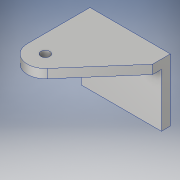
# Autodesk Inventor part: LeftAngleBracket-1111-2018
Saved by Autodesk Inventor 2017 (Build 210142000, 142)
## iProperties
Created: 2018-02-10
Part Number: LeftAngleBracket-1111-2018
Material: Aluminum 6061
Document SubType Name: Modeling
Designer: Phyllis
Density: 2.7 g/cm^3
Appearance: Aluminum - Flat
Author: Phyllis
Autodesk Inventor part; units mm, degrees
ref_plane "YZ Plane" through (0, 0, 0) normal (1, 0, 0) x (0, 1, 0)
ref_plane "XZ Plane" through (0, 0, 0) normal (0, 1, 0) x (-1, 0, 0)
ref_plane "XY Plane" through (0, 0, 0) normal (0, 0, 1) x (1, 0, 0)
sketch "Sketch1" plane through (0, 0, 0) normal (0, 0, 1) x (1, 0, 0)
  line L0 (0, 0) -> (28.575, 0)
  line L1 (28.575, 0) -> (28.575, 19.05)
  line L2 (28.575, 19.05) -> (0, 19.05)
  line L3 (0, 19.05) -> (0, 0)
  dimension "d4" = 28.575
  dimension "d5" = 19.05
  constraints: 8 end point, 2 parallel, 1 horizontal, 1 perpendicular
  measures "d4" distance of L0.start L0.end
  measures "d5" distance of L0.end L1.end
extrude "Extrusion1" add sketch "Sketch1" along normal blind 3.175
sketch "Sketch3" plane through (0, 19.05, 0) normal (0, 1, 0) x (1, 0, 0)
  line L0 (0, 0) -> (28.575, 0) projected
  line L1 (0, 0) -> (28.575, 0)
  line L2 (28.575, 0) -> (28.575, -6.35)
  line L3 (28.575, -6.35) -> (0, -6.35)
  line L4 (0, 0) -> (0, -3.175) projected
  line L5 (0, 0) -> (0, -22.225)
  circle A0 centre (6.35, -22.225) radius 6.35
  line L6 (28.575, -6.35) -> (11.1411, -26.3925)
  circle A1 centre (6.35, -22.225) radius 1.5875
  dimension "d6" = 6.35
  dimension "d8" = 22.225
  dimension "d10" = 28.575
  dimension "d12" = 12.7
  dimension "d13" = 6.35
  dimension "d16" = 3.175
  constraints: 10 end point, 2 centre point, 2 coincident, 2 point on circle, 1 horizontal, 1 parallel, 1 perpendicular, 1 tangent, 1 vertical
  measures "d6" distance between parallel lines of L0 L3
  measures "d8" distance from line of L0 point (6.35, -22.225)
  measures "d10" distance from line of L2 L0.start
  measures "d12" diameter of A0
  measures "d13" horizontal distance of point (6.35, -22.225) L0.start
  measures "d16" diameter of A1
extrude "Extrusion2" add sketch "Sketch3" along normal blind 3.175
body "Solid1"
